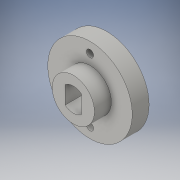
# Autodesk Inventor part: Zoetrope_Motor_Connector v3
Saved by Autodesk Inventor 2016 (Build 200138000, 138)
## iProperties
Created: 2019-01-14
Part Number: Zoetrope_Motor_Connector v3
Material: Generic
Document SubType Name: Modeling
Designer: student
Density: 1 g/cm^3
Appearance: Default
Author: student
Autodesk Inventor part; units mm, degrees
ref_plane "YZ Plane" through (0, 0, 0) normal (1, 0, 0) x (0, 1, 0)
ref_plane "XZ Plane" through (0, 0, 0) normal (0, 1, 0) x (-1, 0, 0)
ref_plane "XY Plane" through (0, 0, 0) normal (0, 0, 1) x (1, 0, 0)
sketch "Sketch1" plane through (0, 0, 0) normal (0, 0, 1) x (1, 0, 0)
  arc A0 (4.953, 6.223) -> (0, 6.223) centre (2.4765, 3.2181) ccw
  arc A1 (0, 0.889) -> (4.953, 0.889) centre (2.4765, 3.8939) ccw
  line L0 (0, 6.223) -> (0, 0.889)
  line L1 (4.953, 6.223) -> (4.953, 0.889)
  circle A2 centre (2.4765, 3.556) radius 6.35
  dimension "d26" = 12.7
  dimension "d27" = 5.334
  dimension "d28" = 4.953
  dimension "d29" = 3.8939
  dimension "d30" = 3.8939
  dimension "d31" = 5.334
  dimension "d32" = 2.794
  dimension "d33" = 0.3379
  dimension "d34" = 2.4765
  dimension "d35" = 2.4765
  constraints: 4 end point, 4 point on circle, 3 centre point, 1 parallel, 1 vertical
  measures "d26" diameter of A2
  measures "d27" distance of L0.start L0.end
  measures "d28" distance between parallel lines of L1 L0
  measures "d29" radius of A0
  measures "d30" radius of A1
  measures "d31" distance of L1.start L1.end
  measures "d33" distance of A1.centre A2.centre
  measures "d34" distance from line of A0.centre L0
  measures "d35" distance from line of A1.centre L0
extrude "Extrusion1" add sketch "Sketch1" along normal blind 5.08
sketch "Sketch2" plane through (2.413, 3.4798, 0) normal (0, 0, -1) x (-1, 0, 0)
  circle A0 centre (0, 0) radius 12.7
  circle A1 centre (0, 0) radius 1.0795
  circle A2 centre (0, 0) radius 6.35 projected
  circle A3 centre (0, 9.525) radius 1.0795
  circle A4 centre (0, -9.525) radius 1.0795
  point P0 (2.413, -3.4798)
  dimension "d16" = 25.4
  dimension "d17" = 2.159
  dimension "d18" = 2.159
  dimension "d19" = 2.159
  constraints: 4 centre point, 1 coincident
  measures "d16" diameter of A0
  measures "d17" diameter of A1
  measures "d18" diameter of A3
  measures "d19" diameter of A4
extrude "Extrusion2" add sketch "Sketch2" along normal blind 5.08 contours A0 | A2
body "Solid1"
